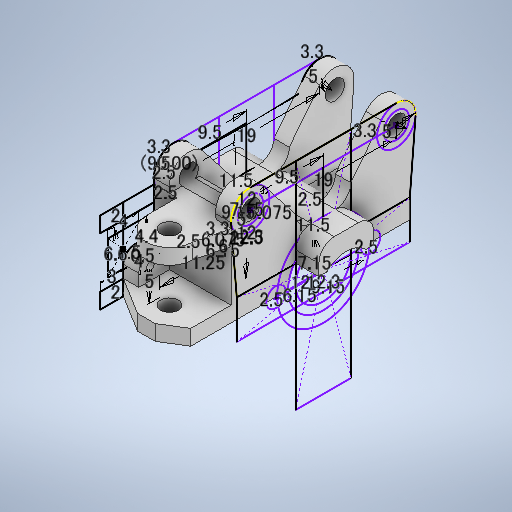
# Autodesk Inventor part: ikafly5.5d_R_2.5
Saved by Autodesk Inventor 2025 (Build 290162000, 162)
## iProperties
Created: 2024-06-20
Part Number: ikafly5.5d_R_2.5
Material: 一般
Document SubType Name: Modeling
Designer: Saigusa
Density: 1 g/cm^3
Appearance: 既定
Author: Saigusa
Autodesk Inventor part; units mm, degrees
ref_plane "YZ Plane" through (0, 0, 0) normal (1, 0, 0) x (0, 1, 0)
ref_plane "XZ Plane" through (0, 0, 0) normal (0, 1, 0) x (-1, 0, 0)
ref_plane "XY Plane" through (0, 0, 0) normal (0, 0, 1) x (1, 0, 0)
sketch "スケッチ1" plane through (0, 0, 0) normal (1, 0, 0) x (0, 1, 0)
  circle A0 centre (0, 0) radius 4.575
  circle A1 centre (0, 0) radius 3.575
  line L0 (0, 0) -> (0, 6)
  line L1 (0, 6) -> (0, -6)
  line L2 (0, 0) -> (11.5, 0)
  line L3 (11.5, 0) -> (11.5, 9.5)
  line L4 (11.5, 9.5) -> (11.5, -9.5)
  circle A2 centre (11.5, 9.5) radius 1.65
  circle A3 centre (11.5, -9.5) radius 1.65
  line L5 (0, 0) -> (0, 11.25)
  line L6 (0, 11.25) -> (0, -11.25)
  line L7 (-2.5, -11.25) -> (2.5, -11.25)
  line L8 (2.5, -11.25) -> (2.5, 11.25)
  line L9 (2.5, 11.25) -> (-2.5, 11.25)
  line L10 (-2.5, 11.25) -> (-2.5, -11.25)
  line L11 (-2.5, -11.25) -> (2.5, 11.25) construction
  line L12 (2.5, -11.25) -> (-2.5, 11.25) construction
  circle A4 centre (11.5, 9.5) radius 2.5
  circle A5 centre (11.5, -9.5) radius 2.5
  line L13 (2.5, 11.25) -> (11.2899, 11.9912)
  line L14 (2.5, -11.25) -> (11.2899, -11.9912)
  line L15 (14, 9.5) -> (14, -9.5)
  line L16 (0, -3.575) -> (14, -3.575)
  line L17 (0, 3.575) -> (14, 3.575)
  circle A6 centre (0, 0) radius 6
  line L18 (0, 0) -> (0, 6.15)
  line L19 (0, 6.15) -> (0, -6.15)
  circle A7 centre (0, 6.15) radius 1.25
  circle A8 centre (0, -6.15) radius 1.25
  line L20 (0, 0) -> (0, -6.075)
  line L21 (0, 0) -> (0, 6.075)
  line L22 (11.5, 9.5) -> (11.5, 12)
  line L23 (11.5, 9.5) -> (14, 9.5) construction
  line L24 (11.5, 12) -> (0, 12)
  line L25 (0, 12) -> (0, 11.25)
  line L26 (0, 12) -> (2, 12)
  line L27 (2, 12) -> (2, 16)
  line L28 (2, 16) -> (0, 16)
  line L29 (0, 16) -> (0, 12)
  line L30 (2, 12) -> (8.6, 12)
  line L31 (8.6, 12) -> (8.6, 16)
  line L32 (8.6, 16) -> (2, 16)
  line L33 (2, 16) -> (2, 12)
  line L34 (8.6, 12) -> (10.6, 12)
  line L35 (10.6, 12) -> (10.6, 16)
  line L36 (10.6, 16) -> (8.6, 16)
  line L37 (8.6, 16) -> (8.6, 12)
  line L38 (0, 16) -> (2, 16)
  line L39 (2, 16) -> (2, 19)
  line L40 (2, 19) -> (0, 19)
  line L41 (0, 19) -> (0, 16)
  line L42 (8.6, 16) -> (10.6, 16)
  line L43 (10.6, 16) -> (10.6, 19)
  line L44 (10.6, 19) -> (8.6, 19)
  line L45 (8.6, 19) -> (8.6, 16)
  line L46 (3.1, 18) -> (7.5, 18)
  line L47 (7.5, 18) -> (7.5, 14)
  line L48 (7.5, 14) -> (3.1, 14)
  line L49 (3.1, 14) -> (3.1, 18)
  line L50 (3.1, 18) -> (7.5, 14) construction
  line L51 (7.5, 18) -> (3.1, 14) construction
  line L52 (3.1, 16) -> (3.6, 16)
  line L53 (3.6, 16) -> (3.6, 14.5)
  line L54 (3.6, 14.5) -> (3.1, 14.5)
  line L55 (3.1, 14.5) -> (3.1, 16)
  circle A9 centre (3.6, 14.5) radius 0.5
  circle A10 centre (3.6, 14.5) radius 1.5
  line L56 (3.6, 14.5) -> (5.1, 14.5)
  line L57 (5.1, 14.5) -> (5.1, 12)
  circle A11 centre (11.5, 9.5) radius 1.25
  line L58 (10.6, 12) -> (10.6, 7.1676)
  line L59 (10.6, 9.5) -> (0, 9.5)
  line L60 (10.6, 8.6325) -> (0, 8.6325)
  line L61 (10.6, 8.1171) -> (0, 8.1171)
  point P0 (0, 4.575)
  point P1 (0, -4.575)
  point P2 (2.5, 3.575)
  point P3 (2.5, 2.5555)
  point P4 (2.5, -2.5555)
  point P5 (2.5, -3.575)
  point P6 (0, 7.4)
  point P7 (0, 4.9)
  point P8 (0, -4.9)
  point P9 (0, -7.4)
  point P10 (2.5, 5.4544)
  point P11 (2.5, -5.4544)
  point P12 (4.8186, 3.575)
  point P13 (4.8186, -3.575)
  point P14 (2.8548, 3.575)
  point P15 (2.8548, -3.575)
  point P16 (5.3, 16)
  point P17 (2.5, 8.1171)
  point P18 (10.6, 10.3675)
  point P19 (5.1, 14)
  point P20 (5.0142, 14)
  dimension "d9" = 3.3
  dimension "d126" = 2.5
  dimension "d0" = 9.15
  dimension "d1" = 7.15
  dimension "d2" = 6
  dimension "d3" = 12
  dimension "d6" = 11.5
  dimension "d7" = 9.5
  dimension "d8" = 19
  dimension "d10" = 3.3
  dimension "d11" = 11.25
  dimension "d12" = 22.5
  dimension "d13" = 5
  dimension "d14" = 5
  dimension "d15" = 5
  dimension "d28" = 12
  dimension "d29" = 6.15
  dimension "d30" = 12.3
  dimension "d31" = 2.5
  dimension "d32" = 2.5
  dimension "d99" = 6.075
  dimension "d100" = 6.075
  dimension "d115" = 2.5
  dimension "d116" = 90
  dimension "d117" = 2
  dimension "d118" = 4
  dimension "d119" = 6.6
  dimension "d120" = 2
  dimension "d121" = 3
  dimension "d122" = 4.4
  dimension "d123" = 4
  dimension "d124" = 0.5
  dimension "d125" = 1.5
  constraints: 124 end point, 22 point on line, 17 parallel, 17 perpendicular, 12 coincident, 10 horizontal, 9 centre point, 9 point on circle, 6 midpoint, 6 tangent, 2 collinear, 1 horizontal alignment, 1 vertical, 8 other
  measures "d0" diameter of A0
  measures "d1" diameter of A1
  measures "d2" distance of L0.start L0.end
  measures "d3" distance of L0.end L1.end
  measures "d6" distance of L0.start L2.end
  measures "d7" distance of L2.end L3.end
  measures "d8" distance of L3.end L4.end
  measures "d10" diameter of A3
  measures "d11" distance of L0.start L5.end
  measures "d12" distance of L5.end L6.end
  measures "d13" distance of L9.end L8.end
  measures "d14" diameter of A4
  measures "d15" diameter of A5
  measures "d28" diameter of A6
  measures "d29" distance of L18.start L18.end
  measures "d30" distance of L18.end L19.end
  measures "d31" diameter of A7
  measures "d32" diameter of A8
  measures "d99" distance of L18.start L20.end
  measures "d100" distance of L18.start L21.end
  measures "d115" distance of L22.start L22.end
  measures "d116" angle of L23 L22
  measures "d117" distance of L28.end L27.end
  measures "d118" distance of L27.end L26.end
  measures "d119" distance of L32.end L31.end
  measures "d120" distance of L36.end L35.end
  measures "d121" distance of L39.end L38.end
  measures "d122" distance of L47.end L48.end
  measures "d123" distance of L46.end L47.end
  measures "d124" distance of L53.end L54.end
  measures "d125" distance of L52.end L53.end
extrude "押し出し7" add sketch "スケッチ1" along normal blind 2 contours L2 A6 L16 A0 | A0 L17 A6 L2 | A0 L8 A6 L17 | L16 A6 L8 A0 | A6 L17 L3 L2 | L2 L4 L16 A6 | A0 L0 A7 A6 L8 | A6 L8 L61 A4 L3 L17 | L8 A6 A8 L1 A0 | L16 L4 A5 L14 L8 A6 | L3 L17 L15 L16 L4 | A6 A7 L5 L61 L8 | L3 A4 L15 L17 | L8 L7 L6 A8 A6 | L16 L15 A5 L4 | L0 A6 A7 | L61 L5 L60 L8 | L8 L60 A4 L61 | A6 L5 A7 | A4 L58 A2 L3 | L3 A2 L22 A4 | A8 A6 L1 | A8 L6 A6 | A5 | L60 L5 L59 L8 | L8 L59 A4 L60 | L61 L58 A4 | A4 L60 A2 L61 | A2 L58 A11 L3 | L3 A11 L22 A2 | L59 L5 L9 L8 | L8 L13 L58 A4 L59 | A4 L59 A2 L60 | A2 L60 L58 | A11 L58 L22 L3 | L3 L22 A11 | L22 A2 L58 A4 | A4 L58 A2 L59 | A2 L59 A11 L60 | A11 L59 L58 | L22 A11 L58 A2 | A4 L58 L13 | A2 L58 A11 L59 | A11 L58 L59 | A3 picked at (0.2292, 5.6392) picked at (0.3961, 6.4211) picked at (0.2292, -5.6392) picked at (0.3961, -6.4211)
extrude "押し出し8" add sketch "スケッチ1" along normal blind 10 contours L2 A6 L16 A0 | A0 L17 A6 L2 | A0 L8 A6 L17 | L16 A6 L8 A0 | A6 L17 L3 L2 | L2 L4 L16 A6 | A0 L0 A7 A6 L8 | L8 A6 A8 L1 A0 | L3 L17 L15 L16 L4 | A6 A7 L5 L61 L8 | L8 L7 L6 A8 A6 | L0 A6 A7 | L61 L5 L60 L8 | A6 L5 A7 | A8 A6 L1 | A8 L6 A6 | L60 L5 L59 L8 | L59 L5 L9 L8 picked at (0.2292, 5.6392) picked at (0.3961, 6.4211) picked at (0.2292, -5.6392) picked at (0.3961, -6.4211)
sketch "スケッチ6" plane through (10, 0, 0) normal (1, 0, 0) x (0, 0, -1)
  line L0 (0, 0) -> (-6.15, 0)
  line L1 (-6.15, 0) -> (6.15, 0)
  circle A0 centre (-6.15, 0) radius 1.25
  circle A1 centre (6.15, 0) radius 1.25
  line L2 (-11.25, 2.5) -> (11.25, 2.5)
  line L3 (11.25, 2.5) -> (11.25, -2.5)
  line L4 (11.25, -2.5) -> (-11.25, -2.5)
  line L5 (-11.25, -2.5) -> (-11.25, 2.5)
  line L6 (-11.25, 2.5) -> (11.25, -2.5) construction
  line L7 (11.25, 2.5) -> (-11.25, -2.5) construction
  line L8 (0, 0) -> (0, 11.5)
  line L9 (0, 11.5) -> (-9.5, 11.5)
  line L10 (-9.5, 11.5) -> (9.5, 11.5)
  circle A2 centre (-9.5, 11.5) radius 1.65
  circle A3 centre (-9.5, 11.5) radius 2.5
  circle A4 centre (9.5, 11.5) radius 1.65
  circle A5 centre (9.5, 11.5) radius 2.5
  circle A6 centre (0, 0) radius 6
  circle A7 centre (0, 0) radius 4.575
  arc A8 (11.9912, 11.2899) -> (9.5, 14) centre (9.5, 11.5) ccw projected
  line L11 (11.25, 2.5) -> (11.9912, 11.2899)
  line L12 (-11.9912, 11.2899) -> (-11.25, 2.5) projected
  line L13 (-11.25, 2.5) -> (-11.9912, 11.2899)
  line L14 (9.5, 14) -> (-9.5, 14) projected
  arc A9 (-9.5, 14) -> (-11.9912, 11.2899) centre (-9.5, 11.5) ccw projected
  line L15 (-9.5, 14) -> (9.5, 14)
  circle A10 centre (0, 0) radius 3.575
  line L16 (-3.575, 14) -> (-3.575, 4.8186) projected
  line L17 (3.575, -14) -> (-3.575, -14)
  line L18 (-3.575, -14) -> (-3.575, 14)
  line L19 (-3.575, 14) -> (3.575, 14)
  line L20 (3.575, 14) -> (3.575, -14)
  line L21 (3.575, -14) -> (-3.575, 14) construction
  line L22 (-3.575, -14) -> (3.575, 14) construction
  point P0 (-5.4544, 2.5)
  point P1 (5.4544, 2.5)
  point P2 (7, 11.5)
  point P3 (-7, 11.5)
  point P4 (-3.575, 11.5)
  point P5 (-3.575, 4.8186)
  point P6 (-3.575, 2.5)
  point P7 (-2.5555, 2.5)
  point P8 (2.5555, 2.5)
  point P9 (3.575, 2.5)
  point P10 (3.575, 11.5)
  dimension "d69" = 12
  dimension "d56" = 6.15
  dimension "d57" = 12.3
  dimension "d58" = 2.5
  dimension "d59" = 2.5
  dimension "d62" = 11.5
  dimension "d63" = 9.5
  dimension "d64" = 19
  dimension "d65" = 3.3
  dimension "d66" = 5
  dimension "d67" = 3.3
  dimension "d68" = 5
  dimension "d70" = 9.15
  dimension "d79" = 7.15
  constraints: 40 end point, 9 coincident, 8 centre point, 5 equal length, 4 horizontal, 4 midpoint, 3 perpendicular, 2 point on line, 2 tangent, 1 vertical, 2 other
  measures "d56" distance of L0.start L0.end
  measures "d57" distance of L0.end L1.end
  measures "d58" diameter of A0
  measures "d59" diameter of A1
  measures "d62" distance of L0.start L8.end
  measures "d63" distance of L8.end L9.end
  measures "d64" distance of L9.end L10.end
  measures "d65" diameter of A2
  measures "d66" diameter of A3
  measures "d67" diameter of A4
  measures "d68" diameter of A5
  measures "d70" diameter of A7
  measures "d79" diameter of A10
extrude "押し出し9" add sketch "スケッチ6" against normal blind 2 contours L2 L12 A3 L9 L16 A6 | L16 L9 L8 A6 | A6 L20 L10 A5 L11 L2 | A6 L8 L10 L20 | L16 L14 L20 L10 L9 | L9 A3 L14 L16 | L20 L14 A5 L10 | A3 | A5 | A2 | A4
extrude "押し出し10" add sketch "スケッチ1" against normal blind 0.5 contours L2 A6 L16 A0 | A0 L17 A6 L2 | A6 L17 L3 L2 | L2 L4 L16 A6 | L3 L17 L15 L16 L4
sketch "スケッチ7" plane through (-0.5, 0, 0) normal (-1, 0, 0) x (0, 0, 1)
  circle A0 centre (0, 0) radius 3.575
  line L0 (-9.5, 14) -> (9.5, 14) projected
  line L1 (-3.575, 14) -> (3.575, 14)
  circle A1 centre (0, 0) radius 4.575
  line L2 (-11.25, 0) -> (-11.25, 2.5) projected
  line L3 (11.25, -2.5) -> (-11.25, -2.5)
  line L4 (-11.25, -2.5) -> (-11.25, 2.5)
  line L5 (-11.25, 2.5) -> (11.25, 2.5)
  line L6 (11.25, 2.5) -> (11.25, -2.5)
  line L7 (11.25, -2.5) -> (-11.25, 2.5) construction
  line L8 (-11.25, -2.5) -> (11.25, 2.5) construction
  line L9 (-3.575, 14) -> (-3.575, 0)
  line L10 (3.575, 14) -> (3.575, 0)
  point P0 (-3.575, 2.5)
  point P1 (-2.5555, 2.5)
  point P2 (2.5555, 2.5)
  point P3 (3.575, 2.5)
  dimension "d75" = 7.15
  dimension "d76" = 5
  constraints: 18 end point, 2 centre point, 2 coincident, 2 midpoint, 2 parallel, 2 point on circle, 2 point on line, 2 tangent, 1 horizontal, 1 perpendicular
  measures "d75" diameter of A0
  measures "d76" distance of L3.end L2.end
extrude "押し出し11" add sketch "スケッチ7" along normal blind 3 contours A0 L5 L9 A1 L10 | A1 L9 L0 L10
extrude "押し出し12" add sketch "スケッチ6" along normal blind 3 contours L2 L18 A7 L8 A10 | A10 L8 A7 L20 L2 | L18 A6 L8 A7 | A7 L8 A6 L20 | L16 L9 L8 A6 | A6 L8 L10 L20 | L16 L14 L20 L10 L9
sketch "スケッチ8" plane through (13, 0, 0) normal (1, 0, 0) x (0, 0, -1)
  line L0 (-3.575, 2.5) -> (-3.575, 14) projected
  line L1 (3.575, 14) -> (3.575, 2.5) projected
  line L2 (-3.575, 14) -> (3.575, 14)
  line L3 (3.575, 14) -> (3.575, 2.5)
  line L4 (3.575, 2.5) -> (-3.575, 2.5)
  line L5 (-3.575, 2.5) -> (-3.575, 14)
  circle A0 centre (0, 0) radius 6
  line L6 (-3.575, 14) -> (3.575, 14)
  line L7 (3.575, 14) -> (3.575, 6)
  line L8 (3.575, 6) -> (-3.575, 6)
  line L9 (-3.575, 6) -> (-3.575, 14)
  dimension "d89" = 12
  constraints: 16 end point, 4 parallel, 2 horizontal, 2 perpendicular, 1 centre point, 1 coincident, 1 point on line
  measures "d89" diameter of A0
extrude "押し出し13" cut sketch "スケッチ8" against normal blind 16.5 contours L0 L2 L1 L8
fillet "フィレット1" radius 2 10 edges at (11.5, 6, -3.575) (11.5, 6, 3.575) (9, 6, 3.575) (9, 6, -3.575) (5, 6, 3.575) (5, 6, -3.575) (1, 6, 3.575) (-1.75, 6, 3.575) (1, 6, -3.575) (-1.75, 6, -3.575)
sketch "スケッチ9" plane through (10, 0, 0) normal (1, 0, 0) x (0, 0, -1)
  arc A0 (2.5555, 2.5) -> (-2.5555, 2.5) centre (0, 0) ccw projected
  line L0 (0, 0) -> (0, 11.5)
  line L1 (0, 11.5) -> (-9.5, 11.5)
  circle A1 centre (9.5, 11.5) radius 1.65 projected
  line L2 (-9.5, 11.5) -> (9.5, 11.5)
  circle A2 centre (-9.5, 11.5) radius 2.5
  circle A3 centre (9.5, 11.5) radius 2.5
  arc A4 (-3.575, 8) -> (-1.575, 6) centre (-1.575, 8) ccw projected
  line L3 (-3.575, 8) -> (-7.5334, 13.0435)
  arc A5 (1.575, 6) -> (3.575, 8) centre (1.575, 8) ccw projected
  line L4 (3.575, 8) -> (7.5334, 13.0435)
  line L5 (9.5, 14) -> (3.575, 14) projected
  line L6 (-3.575, 8) -> (3.575, 8)
  line L7 (3.575, 8) -> (3.575, 14)
  line L8 (3.575, 14) -> (-3.575, 14)
  line L9 (-3.575, 14) -> (-3.575, 8)
  line L10 (-3.575, 8) -> (-9.5, 8)
  line L11 (-9.5, 8) -> (-9.5, 14)
  line L12 (-9.5, 14) -> (-3.575, 14)
  line L13 (-3.575, 14) -> (-3.575, 8)
  line L14 (3.575, 8) -> (9.5, 8)
  line L15 (9.5, 8) -> (9.5, 14)
  line L16 (9.5, 14) -> (3.575, 14)
  line L17 (3.575, 14) -> (3.575, 8)
  dimension "d93" = 11.5
  dimension "d94" = 9.5
  dimension "d95" = 5
  dimension "d96" = 5
  constraints: 34 end point, 6 parallel, 4 perpendicular, 3 horizontal, 3 point on circle, 2 centre point, 2 coincident, 2 tangent, 1 vertical
  measures "d93" distance of L0.start L0.end
  measures "d94" distance of L0.end L1.end
  measures "d95" diameter of A2
  measures "d96" diameter of A3
extrude "押し出し14" cut sketch "スケッチ9" against normal blind 16.5 contours L3 L1 L9 | L7 L2 L4 | L1 L3 A2 L12 L9 | L7 L5 A3 L4 L2
hole "穴2" at (0, 0, -6.075) at (0, 0, 6.075) direction (1, 0, 0) diameter 2.5 depth 2.5
hole "穴3" at (0, 11.5, 9.5) at (0, 11.5, -9.5) direction (1, 0, 0) diameter 2.5 end through all
extrude "押し出し15" add sketch "スケッチ1" along normal blind 10 contours L8 L60 A4 L61 | L8 L59 A4 L60 | A4 L60 A2 L61 | L8 L13 L58 A4 L59 | A4 L59 A2 L60 | A2 L60 L58 | L25 L24 L58 L13 L9 | A4 L58 A2 L59 | A2 L59 A11 L60 | L29 L28 L27 L24 | A2 L58 A11 L59 | L41 L40 L39 L28
extrude "押し出し16" add sketch "スケッチ1" along normal blind 2 contours L27 L32 L49 A10 L48 L57 L24 | L48 A10 L57 | L32 A10 L49 | A10 L49 L48 | L48 A9 L56 A10 | L56 A9 L53 A10 | L53 A9 L49 A10 | L48 L49 A9
sketch "スケッチ10" plane through (0, 0, 4.575) normal (0, -1, 0) x (1, 0, 0)
  line L0 (0, 14.425) -> (0, 2.75) projected
  line L1 (0, 14.425) -> (0, 11.425)
  line L2 (0, 14.425) -> (3, 14.425) construction
  line L3 (0, 11.425) -> (6, 11.425)
  circle A0 centre (6, 11.425) radius 1.15
  line L4 (0, 14.425) -> (10, 14.425) projected
  line L5 (6, 11.425) -> (4.85, 11.425)
  line L6 (4.85, 11.425) -> (4.85, 14.425)
  line L7 (4.85, 14.425) -> (6, 14.425)
  line L8 (6, 14.425) -> (6, 11.425)
  line L9 (0, 11.425) -> (4.85, 14.425)
  line L10 (6, 11.425) -> (7.15, 11.425)
  line L11 (7.15, 11.425) -> (7.15, 14.425)
  line L12 (7.15, 14.425) -> (6, 14.425)
  line L13 (6, 14.425) -> (6, 11.425)
  line L14 (6, 11.425) -> (12, 11.425)
  line L15 (6, 11.425) -> (12, 11.425) construction
  line L16 (12, 11.425) -> (7.15, 14.425)
  line L17 (10, 14.425) -> (10, 0) projected
  line L18 (7.15, 11.425) -> (10, 11.425)
  line L19 (10, 11.425) -> (10, 14.425)
  line L20 (10, 14.425) -> (7.15, 14.425)
  line L21 (7.15, 14.425) -> (7.15, 11.425)
  point P0 (0, -4.575)
  point P1 (10, 12.6621)
  dimension "d131" = 3
  dimension "d132" = 90
  dimension "d133" = 6
  dimension "d134" = 90
  dimension "d135" = 2.3
  dimension "d136" = 6
  dimension "d137" = 0
  constraints: 38 end point, 6 horizontal, 6 parallel, 4 perpendicular, 2 equal length, 2 point on line, 1 centre point, 1 coincident, 1 collinear
  measures "d131" distance of L0.start L1.end
  measures "d132" angle of L1 L2
  measures "d133" distance of L1.end L3.end
  measures "d134" angle of L3 L1
  measures "d135" diameter of A0
  measures "d136" distance of L5.start L14.end
  measures "d137" distance between parallel lines of L14 L15
extrude "押し出し17" cut sketch "スケッチ10" against normal blind 2 contours L4 L9 L0 | A0 L8 L3 | L3 L10 A0 | L8 A0 L10 | L4 L17 L16
sketch "スケッチ11" plane through (0, 10.6, 12) normal (0, 1, 0) x (1, 0, 0)
  line L0 (0, -4) -> (0, 4.675) projected
  line L1 (0, -4) -> (6, -4)
  line L2 (0, -4) -> (6, -4) construction
  circle A0 centre (6, -4) radius 1.15
  circle A1 centre (6, -4) radius 3
  line L3 (2, 0) -> (10, 0) projected
  line L4 (3, -4) -> (9, -4)
  line L5 (9, -4) -> (9, 0)
  line L6 (9, 0) -> (3, 0)
  line L7 (3, 0) -> (3, -4)
  line L8 (9, -4) -> (10, 0)
  line L9 (10, 0) -> (3, 0)
  point P0 (0, 12)
  dimension "d143" = 6
  dimension "d140" = 6
  dimension "d141" = 0
  dimension "d142" = 2.3
  constraints: 16 end point, 3 horizontal, 2 coincident, 2 collinear, 2 parallel, 1 centre point, 1 midpoint, 1 perpendicular, 1 point on line, 3 other
  measures "d140" distance of L0.start L1.end
  measures "d141" distance between parallel lines of L1 L2
  measures "d142" diameter of A0
extrude "押し出し18" add sketch "スケッチ11" against normal blind 2 contours A1 L4 A0 L1 | L7 L3 L5 A1 | L1 A0 L4 A1 | L5 L3 L8
